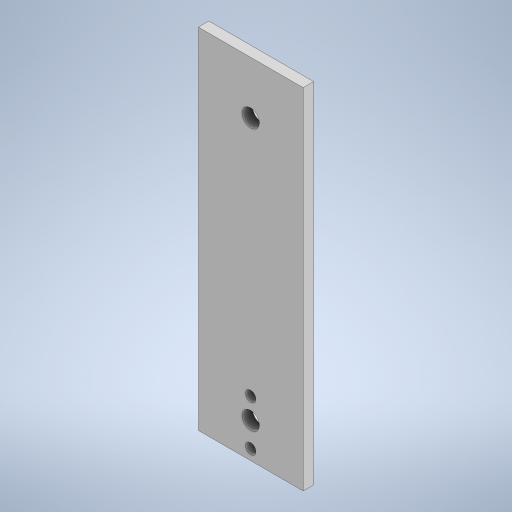
# Autodesk Inventor part: practice_parts02
Saved by Autodesk Inventor 2024.3 (Build 283343000, 343)
## iProperties
Created: 2024-10-22
Part Number: practice_parts02
Material: 一般
Document SubType Name: Modeling
Designer: 佐藤智貴
Density: 1 g/cm^3
Appearance: 既定
Author: 佐藤智貴
Autodesk Inventor part; units mm, degrees
ref_plane "YZ Plane" through (0, 0, 0) normal (1, 0, 0) x (0, 1, 0)
ref_plane "XZ Plane" through (0, 0, 0) normal (0, 1, 0) x (-1, 0, 0)
ref_plane "XY Plane" through (0, 0, 0) normal (0, 0, 1) x (1, 0, 0)
sketch "スケッチ1" plane through (0, 0, 0) normal (0, 0, 1) x (1, 0, 0)
  line L0 (0, 0) -> (30, 0)
  line L1 (30, 0) -> (30, 100)
  line L2 (30, 100) -> (0, 100)
  line L3 (0, 100) -> (0, 0)
  dimension "d0" = 100
  dimension "d1" = 30
  constraints: 8 end point, 2 parallel, 1 horizontal, 1 perpendicular
  measures "d0" distance of L0.end L1.end
  measures "d1" distance of L1.end L2.end
extrude "押し出し1" add sketch "スケッチ1" along normal blind 3
sketch "スケッチ3" plane through (0, 0, 3) normal (0, 0, 1) x (1, 0, 0)
  circle A0 centre (15, 85) radius 2.5
  line L0 (30, 100) -> (0, 100) projected
  line L1 (0, 100) -> (0, 0) projected
  point P0 (15, 100)
  dimension "d9" = 5
  dimension "d10" = 15
  dimension "d11" = 15
  constraints: 1 centre point, 1 midpoint
  measures "d9" diameter of A0
  measures "d10" distance of point (15, 100) A0.centre
  measures "d11" distance from line of L1 A0.centre
extrude "押し出し3" cut sketch "スケッチ3" against normal blind 10
sketch "スケッチ4" plane through (0, 0, 3) normal (0, 0, 1) x (1, 0, 0)
  circle A0 centre (15, 10) radius 2.5
  line L0 (0, 0) -> (30, 0) projected
  line L1 (30, 0) -> (30, 100) projected
  dimension "d14" = 5
  dimension "d15" = 10
  dimension "d16" = 15
  constraints: 1 centre point
  measures "d14" diameter of A0
  measures "d15" distance from line of L0 A0.centre
  measures "d16" distance from line of L1 A0.centre
extrude "押し出し4" cut sketch "スケッチ4" against normal blind 10
sketch "スケッチ5" plane through (0, 0, 3) normal (0, 0, 1) x (1, 0, 0)
  circle A0 centre (15, 10) radius 2.5 projected
  line L0 (15, 10) -> (15, 26.1579)
  line L1 (15, 26.1579) -> (15, -6.7471)
  line L2 (0, 0) -> (30, 0) projected
  point P0 (15, 16)
  point P1 (15, 3)
  dimension "d19" = 3
  dimension "d20" = 13
  constraints: 4 end point, 3 point on line, 1 vertical
  measures "d19" distance from line of L2 point (15, 3)
  measures "d20" distance of point (15, 3) point (15, 16)
hole "穴1" at (15, 16, 3) at (15, 3, 3) direction (0, 0, -1) diameter 3 end through all
equation "\"d11\" = d10"
